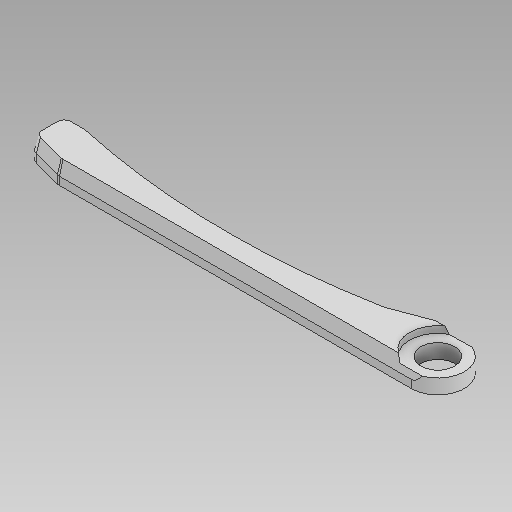
# Autodesk Inventor part: DoubleCrossBar
Saved by Autodesk Inventor 2021 (Build 250183000, 183)
## iProperties
Created: 2021-02-18
Part Number: DoubleCrossBar
Material: 一般
Document SubType Name: Modeling
Designer: kumagai
Density: 1 g/cm^3
Appearance: 既定
Author: kumagai
Autodesk Inventor part; units mm, degrees
ref_plane "YZ Plane" through (0, 0, 0) normal (1, 0, 0) x (0, 1, 0)
ref_plane "XZ Plane" through (0, 0, 0) normal (0, 1, 0) x (-1, 0, 0)
ref_plane "XY Plane" through (0, 0, 0) normal (0, 0, 1) x (1, 0, 0)
sketch "スケッチ1" plane through (0, 0, 0) normal (0, 1, 0) x (-1, 0, 0)
  line L0 (0, -135.4791) -> (0, 27.2465) projected
  line L1 (-16.5662, 0) -> (71.2963, 0) projected
  arc A0 (0, 4) -> (0.0289, -3.9999) centre (0, 0) ccw
  line L2 (0, 4) -> (53.1465, 4)
  arc A1 (55.1096, -2.5) -> (10.5225, -1.6984) centre (30.8359, -112.2326) ccw
  line L3 (58.7446, 2.5) -> (58.7446, -2.5)
  line L4 (0.0289, -3.9999) -> (3.9158, -3.9719)
  circle A2 centre (0, 0) radius 2.55
  line L5 (58.7446, 2.5) -> (53.1465, 4)
  line L6 (58.7446, -2.5) -> (55.1096, -2.5)
  line L7 (3.9158, -3.9719) -> (9.539, -1.8791)
  line L8 (9.539, -1.8791) -> (10.5225, -1.6984)
  dimension "d1" = 8
  dimension "d2" = 116.2326
  dimension "d5" = 5.1
  dimension "d12" = 2.5
  dimension "d13" = 2.5
  dimension "d14" = 15
  dimension "d16" = 58.7446
  dimension "d17" = 27.9086
  dimension "d23" = 20
  dimension "d24" = 1
  dimension "d25" = 10
  dimension "d26" = 6
  dimension "d28" = 112.3852
  constraints: 14 end point, 4 point on circle, 3 centre point, 3 tangent, 2 coincident, 2 horizontal, 1 point on line, 1 vertical
  measures "d1" diameter of A0
  measures "d2" distance from line of A1.centre L2
  measures "d5" diameter of A2
  measures "d12" distance between parallel lines of L6 L1
  measures "d13" distance from line of L1 L3.start
  measures "d14" angle of L2 L5
  measures "d16" distance between parallel lines of L3 L0
  measures "d17" distance from line of A1.centre L3
  measures "d23" angle of L4 L7
  measures "d24" distance of L7.end L8.end
  measures "d25" angle of L7 L8
  measures "d26" distance of L4.end L7.end
  measures "d28" radius of A1
extrude "押し出し1" add sketch "スケッチ1" along normal blind 3.2 contours A0 L1 A2 L0 | L0 A2 L1 A1 L8 L7 L4 A0 | A0 L0 A2 L1 | A2 L0 L2 L5 L3 L1 A1 | L1 L3 L6 A1
fillet "フィレット1" radius 1.5 6 edges at (-58.7446, 1.6, 2.5) (-53.1465, 1.6, 4) (-58.7446, 1.6, -2.5) (-55.1096, 1.6, -2.5) (-3.9158, 1.6, -3.9719) (-9.539, 1.6, -1.8791)
sketch "スケッチ2" plane through (0, 3.2, 0) normal (0, 1, 0) x (1, 0, 0)
  circle A0 centre (0, 0) radius 4.25
  dimension "d9" = 8.5
  constraints: 1 centre point, 1 coincident
  measures "d9" diameter of A0
extrude "押し出し2" cut sketch "スケッチ2" against normal blind 1
chamfer "面取り1" distance 0.5 distance2 2 10 edges at (-27.1926, 3.2, 4) (-53.1448, 3.2, 3.9872) (-55.485, 3.2, 3.3734) (-58.4346, 3.2, 2.2622) (-58.7446, 3.2, 0.1745) (-58.3052, 3.2, -2.0607) (-56.2587, 3.2, -2.5) (-55.111, 3.2, -2.4912) (-32.775, 3.2, 0.136) (-2.5581, 3.2, -3.9816) measured on face at (-58.0379, 3.2, 1.9578) measured on face at (-56.2587, 3.2, -2) measured on face at (-27.1926, 3.2, 3.5) measured on face at (-2.5574, 3.2, -3.8817) measured on face at (-32.7837, 3.2, 0.6359) measured on face at (-58.2446, 3.2, 0.1745) measured on face at (-57.9517, 3.2, -1.7071) measured on face at (-55.3556, 3.2, 2.8904) measured on face at (-55.165, 3.2, -1.9942) measured on face at (-53.0795, 3.2, 3.4914)
